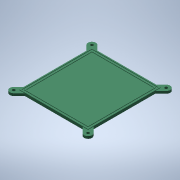
# Autodesk Inventor part: tapa
Saved by Autodesk Inventor 2021 (Build 250183000, 183)
## iProperties
Created: 2021-03-04
Part Number: tapa
Material: Steel, Mild, Welded
Document SubType Name: Modeling
Designer: Usuario
Density: 7.85 g/cm^3
Appearance: Smooth - Dark Sea Green
Author: Usuario
Autodesk Inventor part; units mm, degrees
ref_plane "YZ Plane" through (0, 0, 0) normal (1, 0, 0) x (0, 1, 0)
ref_plane "XZ Plane" through (0, 0, 0) normal (0, 1, 0) x (-1, 0, 0)
ref_plane "XY Plane" through (0, 0, 0) normal (0, 0, 1) x (1, 0, 0)
sketch "Sketch1" plane through (0, 0, 0) normal (0, 1, 0) x (-1, 0, 0)
  line L0 (0, 0) -> (0, -93)
  line L1 (0, -93) -> (88, -93)
  line L2 (88, -93) -> (88, 0)
  line L3 (88, 0) -> (0, 0)
  dimension "d0" = 93
  dimension "d1" = 88
  constraints: 8 end point, 3 perpendicular, 1 vertical
  measures "d0" distance of L0.start L0.end
  measures "d1" distance of L0.end L1.end
extrude "Extrusion1" add sketch "Sketch1" along normal blind 3
sketch "Sketch2" plane through (0, 3, 0) normal (0, 1, 0) x (1, 0, 0)
  line L0 (-88, 93) -> (-88, 0) projected
  line L1 (-88, 0) -> (0, 0)
  line L2 (0, 0) -> (0, 93)
  line L3 (0, 93) -> (-88, 93)
  line L4 (-88, 93) -> (-88, 0)
  line L5 (-88, 0) -> (-88, 1.5)
  line L6 (0, 93) -> (-88, 93) projected
  line L7 (0, 93) -> (0, 91.5)
  line L8 (0, 0) -> (0, 93) projected
  line L9 (-1.5, 91.5) -> (-86.5, 91.5)
  line L10 (-86.5, 91.5) -> (-86.5, 1.5)
  line L11 (-86.5, 1.5) -> (-1.5, 1.5)
  line L12 (-1.5, 1.5) -> (-1.5, 91.5)
  line L13 (-86.5, 1.5) -> (-86.5, 3)
  line L14 (-1.5, 91.5) -> (-1.5, 90)
  line L15 (-85, 3) -> (-3, 3)
  line L16 (-3, 3) -> (-3, 90)
  line L17 (-3, 90) -> (-85, 90)
  line L18 (-85, 90) -> (-85, 3)
  line L19 (-85, 3) -> (-85, 4.5)
  line L20 (-3, 90) -> (-3, 88.5)
  line L21 (-83.5, 4.5) -> (-4.5, 4.5)
  line L22 (-4.5, 4.5) -> (-4.5, 88.5)
  line L23 (-4.5, 88.5) -> (-83.5, 88.5)
  line L24 (-83.5, 88.5) -> (-83.5, 4.5)
  dimension "d4" = 1.5
  dimension "d5" = 1.5
  dimension "d8" = 1.5
  dimension "d11" = 1.5
  dimension "d12" = 1.5
  dimension "d13" = 1.5
  dimension "d15" = 1.5
  constraints: 44 end point, 8 parallel, 6 point on line, 4 horizontal, 4 perpendicular
  measures "d4" distance of L0.end L5.end
  measures "d5" distance of L5.end L10.end
  measures "d8" distance of L10.end L13.end
  measures "d11" distance of L14.end L16.end
  measures "d12" distance of L15.start L19.end
  measures "d13" distance of L19.end L21.start
  measures "d15" distance of L20.end L22.end
extrude "Extrusion2" add sketch "Sketch2" along normal blind 0.7
sketch "Sketch3" plane through (0, 0, 0) normal (0, -1, 0) x (1, 0, 0)
  line L0 (-88, 0) -> (-83, 0) construction
  circle A0 centre (-91.5355, 3.5355) radius 5
  line L1 (-88, 0) -> (0, 0) projected
  line L2 (0, 0) -> (5, 0) construction
  circle A1 centre (3.5355, 3.5355) radius 5
  line L3 (-88, -93) -> (-83, -93) construction
  circle A2 centre (-91.5355, -96.5355) radius 5
  line L4 (0, -93) -> (5, -93) construction
  circle A3 centre (3.5355, -96.5355) radius 5
  line L5 (-86.5, -1.5) -> (-1.5, -1.5) projected
  line L6 (0, -93) -> (-88, -93) projected
  line L7 (0, 0) -> (0, -93) projected
  line L8 (-88, 0) -> (0, 0) projected
  line L9 (-88, -93) -> (-88, 0) projected
  line L10 (-91.5355, 3.5355) -> (-88, 7.0711)
  line L11 (-88, 7.0711) -> (-95.0711, 0)
  line L12 (-95.0711, 0) -> (-88, -7.0711)
  line L13 (-88, -93) -> (-88, 0) projected
  line L14 (-88, 7.0711) -> (-80.9289, 0)
  line L15 (3.5355, 3.5355) -> (7.0711, 7.0711)
  line L16 (7.0711, 7.0711) -> (0, 0)
  line L17 (3.5355, 3.5355) -> (0, 7.0711)
  line L18 (0, 7.0711) -> (-7.0711, 0)
  line L19 (3.5355, 3.5355) -> (7.0711, 0)
  line L20 (7.0711, 0) -> (0, -7.0711)
  line L21 (0, 0) -> (0, -93) projected
  line L22 (-91.5355, -96.5355) -> (-95.0711, -93)
  line L23 (-95.0711, -93) -> (-88, -85.9289)
  line L24 (-91.5355, -96.5355) -> (-88, -100.0711)
  line L25 (-88, -100.0711) -> (-80.9289, -93)
  line L26 (0, -93) -> (-88, -93) projected
  line L27 (3.5355, -96.5355) -> (7.0711, -93)
  line L28 (7.0711, -93) -> (0, -85.9289)
  line L29 (3.5355, -96.5355) -> (0, -100.0711)
  line L30 (0, -100.0711) -> (-7.0711, -93)
  point P0 (-7.0711, -93)
  constraints: 44 end point, 13 point on circle, 12 point on line, 8 perpendicular, 4 centre point, 4 horizontal, 4 tangent, 1 collinear, 1 parallel
extrude "Extrusion3" add sketch "Sketch3" against normal blind 3 contours A0 L11 L10 | A0 L14 L1 | L10 L11 A0 | L9 L12 A0 | L18 A1 L1 | L9 A2 L23 | L16 L19 A1 | A1 L20 L7 | A1 L17 L16 | A1 L15 L17 | L6 L25 A2 | A2 L24 L22 | L22 L24 A2 | L19 L15 A1 | L28 A3 L7 | L6 A3 L30 | A3 L27 L29 | A3 L29 L27
sketch "Sketch4" plane through (0, 0, 0) normal (0, -1, 0) x (1, 0, 0)
  line L0 (0, -7.0711) -> (0, -85.9289) projected
  line L1 (0, -7.0711) -> (7.0711, 0) projected
  arc A0 (7.0711, 0) -> (0, 7.0711) centre (3.5355, 3.5355) ccw projected
  line L2 (0, 7.0711) -> (-7.0711, 0) projected
  line L3 (-80.9289, 0) -> (-7.0711, 0) projected
  line L4 (-80.9289, 0) -> (-88, 7.0711) projected
  arc A1 (-88, 7.0711) -> (-95.0711, 0) centre (-91.5355, 3.5355) ccw projected
  line L5 (-95.0711, 0) -> (-88, -7.0711) projected
  line L6 (-88, -85.9289) -> (-88, -7.0711) projected
  line L7 (-88, -85.9289) -> (-95.0711, -93) projected
  arc A2 (-95.0711, -93) -> (-88, -100.0711) centre (-91.5355, -96.5355) ccw projected
  line L8 (-88, -100.0711) -> (-80.9289, -93) projected
  line L9 (-7.0711, -93) -> (-80.9289, -93) projected
  line L10 (-7.0711, -93) -> (0, -100.0711) projected
  arc A3 (0, -100.0711) -> (7.0711, -93) centre (3.5355, -96.5355) ccw projected
  line L11 (7.0711, -93) -> (0, -85.9289) projected
  arc A4 (-88, 7.0711) -> (-95.0711, 0) centre (-91.5355, 3.5355) ccw projected
  circle A5 centre (-91.5355, 3.5355) radius 1.75
  circle A6 centre (3.5355, 3.5355) radius 1.75
  circle A7 centre (-91.5355, -96.5355) radius 1.75
  circle A8 centre (3.5355, -96.5355) radius 1.75
  point P0 (0, 0)
  dimension "d28" = 3.5
  dimension "d29" = 3.5
  dimension "d30" = 3.5
  dimension "d31" = 3.5
  constraints: 4 centre point, 4 coincident
  measures "d28" diameter of A5
  measures "d29" diameter of A6
  measures "d30" diameter of A7
  measures "d31" diameter of A8
extrude "Extrusion4" cut sketch "Sketch4" against normal blind 3 contours A5 | A6 | A7 | A8
sketch "Sketch5" plane through (0, 0, 0) normal (0, -1, 0) x (1, 0, 0)
  line L0 (-66.5065, -39.4561) -> (-11.1351, -39.4561) construction
  line L1 (-11.1351, -39.4561) -> (-11.1351, -52.4445) construction
  line L2 (-11.1351, -52.4445) -> (-66.5065, -52.4445) construction
  line L3 (-66.5065, -52.4445) -> (-66.5065, -39.4561) construction
  line L4 (-59.6994, -49.4561) -> (-65.4936, -49.4561)
  line L5 (-65.4936, -49.4561) -> (-65.4936, -39.4561)
  line L6 (-65.4936, -39.4561) -> (-64.1646, -39.4561)
  line L7 (-64.1646, -39.4561) -> (-64.1646, -48.273)
  line L8 (-64.1646, -48.273) -> (-59.6994, -48.273)
  line L9 (-59.6994, -48.273) -> (-59.6994, -49.4561)
  line L10 (-55.1694, -49.4561) -> (-59.043, -49.4561)
  line L11 (-59.043, -49.4561) -> (-59.043, -48.4351)
  line L12 (-59.043, -48.4351) -> (-57.7707, -48.4351)
  line L13 (-57.7707, -48.4351) -> (-57.7707, -40.4772)
  line L14 (-57.7707, -40.4772) -> (-59.043, -40.4772)
  line L15 (-59.043, -40.4772) -> (-59.043, -39.4561)
  line L16 (-59.043, -39.4561) -> (-55.1694, -39.4561)
  line L17 (-55.1694, -39.4561) -> (-55.1694, -40.4772)
  line L18 (-55.1694, -40.4772) -> (-56.4417, -40.4772)
  line L19 (-56.4417, -40.4772) -> (-56.4417, -48.4351)
  line L20 (-56.4417, -48.4351) -> (-55.1694, -48.4351)
  line L21 (-55.1694, -48.4351) -> (-55.1694, -49.4561)
  line L22 (-46.3688, -49.4561) -> (-47.8599, -49.4561)
  line L23 (-47.8599, -49.4561) -> (-52.2845, -40.8338)
  line L24 (-52.2845, -40.8338) -> (-52.2845, -49.4561)
  line L25 (-52.2845, -49.4561) -> (-53.5244, -49.4561)
  line L26 (-53.5244, -49.4561) -> (-53.5244, -39.4561)
  line L27 (-53.5244, -39.4561) -> (-51.6362, -39.4561)
  line L28 (-51.6362, -39.4561) -> (-47.6086, -47.3735)
  line L29 (-47.6086, -47.3735) -> (-47.6086, -39.4561)
  line L30 (-47.6086, -39.4561) -> (-46.3688, -39.4561)
  line L31 (-46.3688, -39.4561) -> (-46.3688, -49.4561)
  line L32 (-37.0495, -49.4561) -> (-38.7756, -49.4561)
  line L33 (-38.7756, -49.4561) -> (-42.4304, -44.8046)
  line L34 (-42.4304, -44.8046) -> (-43.0138, -45.461)
  line L35 (-43.0138, -45.461) -> (-43.0138, -49.4561)
  line L36 (-43.0138, -49.4561) -> (-44.3428, -49.4561)
  line L37 (-44.3428, -49.4561) -> (-44.3428, -39.4561)
  line L38 (-44.3428, -39.4561) -> (-43.0138, -39.4561)
  line L39 (-43.0138, -39.4561) -> (-43.0138, -44.0509)
  line L40 (-43.0138, -44.0509) -> (-38.9133, -39.4561)
  line L41 (-38.9133, -39.4561) -> (-37.2926, -39.4561)
  line L42 (-37.2926, -39.4561) -> (-41.4336, -43.9213)
  line L43 (-41.4336, -43.9213) -> (-37.0495, -49.4561)
  line L44 (-36.2553, -49.4561) -> (-36.2553, -39.4561)
  line L45 (-36.2553, -39.4561) -> (-29.9992, -39.4561)
  line L46 (-29.9992, -39.4561) -> (-29.9992, -40.6393)
  line L47 (-29.9992, -40.6393) -> (-34.9263, -40.6393)
  line L48 (-34.9263, -40.6393) -> (-34.9263, -43.3783)
  line L49 (-34.9263, -43.3783) -> (-30.3315, -43.3783)
  line L50 (-30.3315, -43.3783) -> (-30.3315, -44.5615)
  line L51 (-30.3315, -44.5615) -> (-34.9263, -44.5615)
  line L52 (-34.9263, -44.5615) -> (-34.9263, -48.273)
  line L53 (-34.9263, -48.273) -> (-29.9992, -48.273)
  line L54 (-29.9992, -48.273) -> (-29.9992, -49.4561)
  line L55 (-29.9992, -49.4561) -> (-36.2553, -49.4561)
  line L56 (-20.8015, -49.4561) -> (-22.5276, -49.4561)
  line L57 (-22.5276, -49.4561) -> (-25.6881, -45.4772)
  line L58 (-25.6881, -45.4772) -> (-27.2116, -45.4772)
  line L59 (-27.2116, -45.4772) -> (-27.2116, -49.4561)
  line L60 (-27.2116, -49.4561) -> (-28.5406, -49.4561)
  line L61 (-28.5406, -49.4561) -> (-28.5406, -39.4561)
  line L62 (-28.5406, -39.4561) -> (-25.9636, -39.4561)
  spline S0 degree 2 poles (-25.9636, -39.4561) (-25.1046, -39.4561) (-23.9458, -39.6425) (-23.419, -39.9829) knots 0 0 0 1 2 2 2
  spline S1 degree 2 poles (-23.419, -39.9829) (-22.8923, -40.3232) (-22.2845, -41.3848) (-22.2845, -42.1709) knots 0 0 0 1 2 2 2
  spline S2 degree 2 poles (-22.2845, -42.1709) (-22.2845, -43.2649) (-23.4028, -44.7479) (-24.359, -45.1044) knots 0 0 0 1 2 2 2
  line L63 (-24.359, -45.1044) -> (-20.8015, -49.4561)
  spline S3 degree 2 poles (-23.6702, -42.2762) (-23.6702, -41.8386) (-23.9782, -41.166) (-24.3023, -40.9472) knots 0 0 0 1 2 2 2
  spline S4 degree 2 poles (-24.3023, -40.9472) (-24.5859, -40.7608) (-25.3396, -40.6069) (-25.8906, -40.6069) knots 0 0 0 1 2 2 2
  line L64 (-25.8906, -40.6069) -> (-27.2116, -40.6069)
  line L65 (-27.2116, -40.6069) -> (-27.2116, -44.367)
  line L66 (-27.2116, -44.367) -> (-26.0446, -44.367)
  spline S5 degree 2 poles (-26.0446, -44.367) (-25.4693, -44.367) (-24.5535, -44.1644) (-24.2375, -43.8484) knots 0 0 0 1 2 2 2
  spline S6 degree 2 poles (-24.2375, -43.8484) (-23.9458, -43.5728) (-23.6702, -42.7949) (-23.6702, -42.2762) knots 0 0 0 1 2 2 2
  point P0 (0, 0)
  constraints: 2 other
extrude "Extrusion5" cut sketch "Sketch5" against normal blind 1
body "Solid1"
